Autodesk Inventor part; units mm, degrees
(part 4 of 6)
sketch "スケッチ4" plane through (0, 0, 3) normal (0, 0, 1) x (1, 0, 0)
  circle A0 centre (148.5, 105) radius 2 projected
  arc A1 (148.9109, 125.0429) -> (148.7771, 124.6719) centre (154.869, 122.6849) ccw projected
  arc A2 (149.1052, 125.4911) -> (148.9109, 125.0429) centre (155.9658, 122.2508) ccw projected
  arc A3 (149.5044, 125.4754) -> (149.1052, 125.4911) centre (148.5, 105) ccw projected
  arc A4 (149.6629, 125.0133) -> (149.5044, 125.4754) centre (142.4106, 122.7834) ccw projected
  arc A5 (149.7671, 124.633) -> (149.6629, 125.0133) centre (143.5382, 123.1301) ccw projected
  arc A6 (149.831, 124.3292) -> (149.7671, 124.633) centre (144.6423, 123.3965) ccw projected
  arc A7 (150.2091, 124.2995) -> (149.831, 124.3292) centre (148.5, 105) ccw projected
  arc A8 (150.3197, 124.5895) -> (150.2091, 124.2995) centre (155.1881, 122.5665) ccw projected
  arc A9 (150.4822, 124.9489) -> (150.3197, 124.5895) centre (156.2369, 122.1307) ccw projected
  arc A10 (150.7111, 125.3804) -> (150.4822, 124.9489) centre (157.2963, 121.6119) ccw projected
  arc A11 (151.1078, 125.3335) -> (150.7111, 125.3804) centre (148.5, 105) ccw projected
  arc A12 (151.2295, 124.8604) -> (151.1078, 125.3335) centre (143.8247, 123.2064) ccw projected
  arc A13 (151.3036, 124.473) -> (151.2295, 124.8604) centre (144.9759, 123.4635) ccw projected
  arc A14 (151.3435, 124.1652) -> (151.3036, 124.473) centre (146.0975, 123.6425) ccw projected
  arc A15 (151.7181, 124.1059) -> (151.3435, 124.1652) centre (148.5, 105) ccw projected
  arc A16 (151.8511, 124.3863) -> (151.7181, 124.1059) centre (156.5457, 121.9876) ccw projected
  arc A17 (152.0413, 124.7318) -> (151.8511, 124.3863) centre (157.5571, 121.4708) ccw projected
  arc A18 (152.3033, 125.1441) -> (152.0413, 124.7318) centre (158.5726, 120.8705) ccw projected
  arc A19 (152.6951, 125.0662) -> (152.3033, 125.1441) centre (148.5, 105) ccw projected
  arc A20 (152.7793, 124.585) -> (152.6951, 125.0662) centre (145.2676, 123.517) ccw projected
  arc A21 (152.8228, 124.193) -> (152.7793, 124.585) centre (146.4354, 123.6831) ccw projected
  arc A22 (152.8384, 123.883) -> (152.8228, 124.193) centre (147.5676, 123.7735) ccw projected
  arc A23 (153.2072, 123.7945) -> (152.8384, 123.883) centre (148.5, 105) ccw projected
  arc A24 (153.3618, 124.0636) -> (153.2072, 123.7945) centre (157.8537, 121.304) ccw projected
  arc A25 (153.5785, 124.3932) -> (153.3618, 124.0636) centre (158.8215, 120.7095) ccw projected
  arc A26 (153.872, 124.7836) -> (153.5785, 124.3932) centre (159.7867, 120.0313) ccw projected
  arc A27 (154.2565, 124.6752) -> (153.872, 124.7836) centre (148.5, 105) ccw projected
  arc A28 (154.3028, 124.1889) -> (154.2565, 124.6752) centre (146.7304, 123.7136) ccw projected
  arc A29 (154.3154, 123.7947) -> (154.3028, 124.1889) centre (147.9076, 123.7875) ccw projected
  arc A30 (154.3066, 123.4844) -> (154.3154, 123.7947) centre (149.0434, 123.7888) ccw projected
  arc A31 (154.6673, 123.3672) -> (154.3066, 123.4844) centre (148.5, 105) ccw projected
  arc A32 (154.8425, 123.6234) -> (154.6673, 123.3672) centre (159.1041, 120.5199) ccw projected
  arc A33 (155.0844, 123.9349) -> (154.8425, 123.6234) centre (160.0222, 119.8512) ccw projected
  arc A34 (155.4077, 124.3011) -> (155.0844, 123.9349) centre (160.9312, 119.0994) ccw projected
  arc A35 (155.7825, 124.1629) -> (155.4077, 124.3011) centre (148.5, 105) ccw projected
  arc A36 (155.7904, 123.6745) -> (155.7825, 124.1629) centre (148.2041, 123.7947) ccw projected
  arc A37 (155.772, 123.2805) -> (155.7904, 123.6745) centre (149.3835, 123.776) ccw projected
  arc A38 (155.7389, 122.9719) -> (155.772, 123.2805) centre (150.5159, 123.6882) ccw projected
  arc A39 (156.0893, 122.8267) -> (155.7389, 122.9719) centre (148.5, 105) ccw projected
  arc A40 (156.2842, 123.0684) -> (156.0893, 122.8267) centre (160.2891, 119.64) ccw projected
  arc A41 (156.5497, 123.36) -> (156.2842, 123.0684) centre (161.1519, 118.9014) ccw projected
  arc A42 (156.9007, 123.6997) -> (156.5497, 123.36) centre (161.9991, 118.0806) ccw projected
  arc A43 (157.2635, 123.5324) -> (156.9007, 123.6997) centre (148.5, 105) ccw projected
  arc A44 (157.2331, 123.0449) -> (157.2635, 123.5324) centre (149.6796, 123.76) ccw projected
  arc A45 (157.1839, 122.6536) -> (157.2331, 123.0449) centre (150.8539, 123.6488) ccw projected
  arc A46 (157.1267, 122.3485) -> (157.1839, 122.6536) centre (151.976, 123.4724) ccw projected
  arc A47 (157.4646, 122.1763) -> (157.1267, 122.3485) centre (148.5, 105) ccw projected
  arc A48 (157.6778, 122.4019) -> (157.4646, 122.1763) centre (161.4014, 118.6699) ccw projected
  arc A49 (157.9654, 122.6718) -> (157.6778, 122.4019) centre (162.2036, 117.8659) ccw projected
  arc A50 (158.342, 122.9829) -> (157.9654, 122.6718) centre (162.9838, 116.9812) ccw projected
  arc A51 (158.6905, 122.7877) -> (158.342, 122.9829) centre (148.5, 105) ccw projected
  arc A52 (158.622, 122.3041) -> (158.6905, 122.7877) centre (151.1478, 123.6096) ccw projected
  arc A53 (158.5422, 121.9178) -> (158.622, 122.3041) centre (152.3099, 123.4067) ccw projected
  arc A54 (158.4612, 121.6182) -> (158.5422, 121.9178) centre (153.4146, 123.1428) ccw projected
  arc A55 (158.7846, 121.42) -> (158.4612, 121.6182) centre (148.5, 105) ccw projected
  arc A56 (159.0148, 121.6282) -> (158.7846, 121.42) centre (162.4341, 117.6156) ccw projected
  arc A57 (159.3227, 121.8747) -> (159.0148, 121.6282) centre (163.1708, 116.7511) ccw projected
  arc A58 (159.7226, 122.1553) -> (159.3227, 121.8747) centre (163.8792, 115.8078) ccw projected
  arc A59 (160.0547, 121.9334) -> (159.7226, 122.1553) centre (148.5, 105) ccw projected
  arc A60 (159.9485, 121.4566) -> (160.0547, 121.9334) centre (152.5998, 123.3445) ccw projected
  arc A61 (159.8386, 121.0778) -> (159.9485, 121.4566) centre (153.7423, 123.051) ccw projected
  arc A62 (159.7344, 120.7854) -> (159.8386, 121.0778) centre (154.8229, 122.7012) ccw projected
  arc A63 (160.0412, 120.5625) -> (159.7344, 120.7854) centre (148.5, 105) ccw projected
  arc A64 (160.2871, 120.752) -> (160.0412, 120.5625) centre (163.381, 116.4834) ccw projected
  arc A65 (160.6134, 120.9735) -> (160.2871, 120.752) centre (164.0476, 115.5638) ccw projected
  arc A66 (161.034, 121.2219) -> (160.6134, 120.9735) centre (164.6798, 114.5679) ccw projected
  arc A67 (161.3477, 120.9746) -> (161.034, 121.2219) centre (148.5, 105) ccw projected
  arc A68 (161.2043, 120.5076) -> (161.3477, 120.9746) centre (154.0264, 122.9663) ccw projected
  arc A69 (161.0651, 120.1386) -> (161.2043, 120.5076) centre (155.1424, 122.5841) ccw projected
  arc A70 (160.9383, 119.8553) -> (161.0651, 120.1386) centre (156.1922, 122.1506) ccw projected
  arc A71 (161.2266, 119.609) -> (160.9383, 119.8553) centre (148.5, 105) ccw projected
  arc A72 (161.4866, 119.7786) -> (161.2266, 119.609) centre (164.2361, 115.2805) ccw projected
  arc A73 (161.8293, 119.9739) -> (161.4866, 119.7786) centre (164.8285, 114.3114) ccw projected
  arc A74 (162.2681, 120.1885) -> (161.8293, 119.9739) centre (165.3806, 113.2689) ccw projected
  arc A75 (162.5614, 119.9173) -> (162.2681, 120.1885) centre (148.5, 105) ccw projected
  arc A76 (162.3819, 119.463) -> (162.5614, 119.9173) centre (155.419, 122.4773) ccw projected
  arc A77 (162.2141, 119.1061) -> (162.3819, 119.463) centre (156.5015, 122.0087) ccw projected
  arc A78 (162.0655, 118.8336) -> (162.2141, 119.1061) centre (157.5141, 121.4942) ccw projected
  arc A79 (162.3336, 118.5655) -> (162.0655, 118.8336) centre (148.5, 105) ccw projected
  arc A80 (162.6061, 118.7141) -> (162.3336, 118.5655) centre (164.9942, 114.0141) ccw projected
  arc A81 (162.963, 118.8819) -> (162.6061, 118.7141) centre (165.5087, 113.0015) ccw projected
  arc A82 (163.4173, 119.0614) -> (162.963, 118.8819) centre (165.9773, 111.919) ccw projected
  arc A83 (163.6885, 118.7681) -> (163.4173, 119.0614) centre (148.5, 105) ccw projected
  arc A84 (163.4738, 118.3293) -> (163.6885, 118.7681) centre (156.7689, 121.8806) ccw projected
  arc A85 (163.2786, 117.9866) -> (163.4738, 118.3293) centre (157.8114, 121.3285) ccw projected
  arc A86 (163.109, 117.7266) -> (163.2786, 117.9866) centre (158.7805, 120.7361) ccw projected
  arc A87 (163.3553, 117.4383) -> (163.109, 117.7266) centre (148.5, 105) ccw projected
  arc A88 (163.6386, 117.5651) -> (163.3553, 117.4383) centre (165.6506, 112.6922) ccw projected
  arc A89 (164.0076, 117.7043) -> (163.6386, 117.5651) centre (166.0841, 111.6424) ccw projected
  arc A90 (164.4746, 117.8477) -> (164.0076, 117.7043) centre (166.4663, 110.5264) ccw projected
  arc A91 (164.7219, 117.534) -> (164.4746, 117.8477) centre (148.5, 105) ccw projected
  arc A92 (164.4735, 117.1134) -> (164.7219, 117.534) centre (158.0679, 121.1798) ccw projected
  arc A93 (164.252, 116.7871) -> (164.4735, 117.1134) centre (159.0638, 120.5476) ccw projected
  arc A94 (164.0625, 116.5412) -> (164.252, 116.7871) centre (159.9834, 119.881) ccw projected
  arc A95 (164.2854, 116.2344) -> (164.0625, 116.5412) centre (148.5, 105) ccw projected
  arc A96 (164.5778, 116.3386) -> (164.2854, 116.2344) centre (166.2012, 111.3229) ccw projected
  arc A97 (164.9566, 116.4485) -> (164.5778, 116.3386) centre (166.551, 110.2423) ccw projected
  arc A98 (165.4334, 116.5547) -> (164.9566, 116.4485) centre (166.8445, 109.0998) ccw projected
  arc A99 (165.6553, 116.2226) -> (165.4334, 116.5547) centre (148.5, 105) ccw projected
  arc A100 (165.3747, 115.8227) -> (165.6553, 116.2226) centre (159.3078, 120.3792) ccw projected
  arc A101 (165.1282, 115.5148) -> (165.3747, 115.8227) centre (160.2511, 119.6708) ccw projected
  arc A102 (164.92, 115.2846) -> (165.1282, 115.5148) centre (161.1156, 118.9341) ccw projected
  arc A103 (165.1182, 114.9612) -> (164.92, 115.2846) centre (148.5, 105) ccw projected
  arc A104 (165.4178, 115.0422) -> (165.1182, 114.9612) centre (166.6428, 109.9146) ccw projected
  arc A105 (165.8041, 115.122) -> (165.4178, 115.0422) centre (166.9067, 108.8099) ccw projected
  arc A106 (166.2877, 115.1905) -> (165.8041, 115.122) centre (167.1096, 107.6478) ccw projected
  arc A107 (166.4829, 114.842) -> (166.2877, 115.1905) centre (148.5, 105) ccw projected
  arc A108 (166.1718, 114.4654) -> (166.4829, 114.842) centre (160.4812, 119.4838) ccw projected
  arc A109 (165.9019, 114.1778) -> (166.1718, 114.4654) centre (161.3659, 118.7036) ccw projected
  arc A110 (165.6763, 113.9646) -> (165.9019, 114.1778) centre (162.1699, 117.9014) ccw projected
  arc A111 (165.8485, 113.6267) -> (165.6763, 113.9646) centre (148.5, 105) ccw projected
  arc A112 (166.1536, 113.6839) -> (165.8485, 113.6267) centre (166.9724, 108.476) ccw projected
  arc A113 (166.5449, 113.7331) -> (166.1536, 113.6839) centre (167.1488, 107.3539) ccw projected
  arc A114 (167.0324, 113.7635) -> (166.5449, 113.7331) centre (167.26, 106.1796) ccw projected
  arc A115 (167.1997, 113.4007) -> (167.0324, 113.7635) centre (148.5, 105) ccw projected
  arc A116 (166.86, 113.0497) -> (167.1997, 113.4007) centre (161.5806, 118.4991) ccw projected
  arc A117 (166.5684, 112.7842) -> (166.86, 113.0497) centre (162.4014, 117.6519) ccw projected
  arc A118 (166.3267, 112.5893) -> (166.5684, 112.7842) centre (163.14, 116.7891) ccw projected
  arc A119 (166.4719, 112.2389) -> (166.3267, 112.5893) centre (148.5, 105) ccw projected
  arc A120 (166.7805, 112.272) -> (166.4719, 112.2389) centre (167.1882, 107.0159) ccw projected
  arc A121 (167.1745, 112.2904) -> (166.7805, 112.272) centre (167.276, 105.8835) ccw projected
  arc A122 (167.6629, 112.2825) -> (167.1745, 112.2904) centre (167.2947, 104.7041) ccw projected
  arc A123 (167.8011, 111.9077) -> (167.6629, 112.2825) centre (148.5, 105) ccw projected
  arc A124 (167.4349, 111.5844) -> (167.8011, 111.9077) centre (162.5994, 117.4312) ccw projected
  arc A125 (167.1234, 111.3425) -> (167.4349, 111.5844) centre (163.3512, 116.5222) ccw projected
  arc A126 (166.8672, 111.1673) -> (167.1234, 111.3425) centre (164.0199, 115.6041) ccw projected
  arc A127 (166.9844, 110.8066) -> (166.8672, 111.1673) centre (148.5, 105) ccw projected
  arc A128 (167.2947, 110.8154) -> (166.9844, 110.8066) centre (167.2888, 105.5434) ccw projected
  arc A129 (167.6889, 110.8028) -> (167.2947, 110.8154) centre (167.2875, 104.4076) ccw projected
  arc A130 (168.1752, 110.7565) -> (167.6889, 110.8028) centre (167.2136, 103.2304) ccw projected
  arc A131 (168.2836, 110.372) -> (168.1752, 110.7565) centre (148.5, 105) ccw projected
  arc A132 (167.8932, 110.0785) -> (168.2836, 110.372) centre (163.5313, 116.2867) ccw projected
  arc A133 (167.5636, 109.8618) -> (167.8932, 110.0785) centre (164.2095, 115.3215) ccw projected
  arc A134 (167.2945, 109.7072) -> (167.5636, 109.8618) centre (164.804, 114.3537) ccw projected
  arc A135 (167.383, 109.3384) -> (167.2945, 109.7072) centre (148.5, 105) ccw projected
  arc A136 (167.693, 109.3228) -> (167.383, 109.3384) centre (167.2735, 104.0676) ccw projected
  arc A137 (168.085, 109.2793) -> (167.693, 109.3228) centre (167.1831, 102.9354) ccw projected
  arc A138 (168.5662, 109.1951) -> (168.085, 109.2793) centre (167.017, 101.7676) ccw projected
  arc A139 (168.6441, 108.8033) -> (168.5662, 109.1951) centre (148.5, 105) ccw projected
  arc A140 (168.2318, 108.5413) -> (168.6441, 108.8033) centre (164.3705, 115.0726) ccw projected
  arc A141 (167.8863, 108.3511) -> (168.2318, 108.5413) centre (164.9708, 114.0571) ccw projected
  arc A142 (167.6059, 108.2181) -> (167.8863, 108.3511) centre (165.4876, 113.0457) ccw projected
  arc A143 (167.6652, 107.8435) -> (167.6059, 108.2181) centre (148.5, 105) ccw projected
  arc A144 (167.973, 107.8036) -> (167.6652, 107.8435) centre (167.1425, 102.5975) ccw projected
  arc A145 (168.3604, 107.7295) -> (167.973, 107.8036) centre (166.9635, 101.4759) ccw projected
  arc A146 (168.8335, 107.6078) -> (168.3604, 107.7295) centre (166.7064, 100.3247) ccw projected
  arc A147 (168.8804, 107.2111) -> (168.8335, 107.6078) centre (148.5, 105) ccw projected
  arc A148 (168.4489, 106.9822) -> (168.8804, 107.2111) centre (165.1119, 113.7963) ccw projected
  arc A149 (168.0895, 106.8197) -> (168.4489, 106.9822) centre (165.6307, 112.7369) ccw projected
  arc A150 (167.7995, 106.7091) -> (168.0895, 106.8197) centre (166.0665, 111.6881) ccw projected
  arc A151 (167.8292, 106.331) -> (167.7995, 106.7091) centre (148.5, 105) ccw projected
  arc A152 (168.133, 106.2671) -> (167.8292, 106.331) centre (166.8965, 101.1423) ccw projected
  arc A153 (168.5133, 106.1629) -> (168.133, 106.2671) centre (166.6301, 100.0382) ccw projected
  arc A154 (168.9754, 106.0044) -> (168.5133, 106.1629) centre (166.2834, 98.9106) ccw projected
  arc A155 (168.9911, 105.6052) -> (168.9754, 106.0044) centre (148.5, 105) ccw projected
  arc A156 (168.5429, 105.4109) -> (168.9911, 105.6052) centre (165.7508, 112.4658) ccw projected
  arc A157 (168.1719, 105.2771) -> (168.5429, 105.4109) centre (166.1849, 111.369) ccw projected
  arc A158 (167.8741, 105.1896) -> (168.1719, 105.2771) centre (166.5371, 110.2892) ccw projected
  arc A159 (167.8741, 104.8104) -> (167.8741, 105.1896) centre (148.5, 105) ccw projected
  arc A160 (168.1719, 104.7229) -> (167.8741, 104.8104) centre (166.5371, 99.7108) ccw projected
  arc A161 (168.5429, 104.5891) -> (168.1719, 104.7229) centre (166.1849, 98.631) ccw projected
  arc A162 (168.9911, 104.3948) -> (168.5429, 104.5891) centre (165.7508, 97.5342) ccw projected
  arc A163 (168.9754, 103.9956) -> (168.9911, 104.3948) centre (148.5, 105) ccw projected
  arc A164 (168.5133, 103.8371) -> (168.9754, 103.9956) centre (166.2834, 111.0894) ccw projected
  arc A165 (168.133, 103.7329) -> (168.5133, 103.8371) centre (166.6301, 109.9618) ccw projected
  arc A166 (167.8292, 103.669) -> (168.133, 103.7329) centre (166.8965, 108.8577) ccw projected
  arc A167 (167.7995, 103.2909) -> (167.8292, 103.669) centre (148.5, 105) ccw projected
  arc A168 (168.0895, 103.1803) -> (167.7995, 103.2909) centre (166.0665, 98.3119) ccw projected
  arc A169 (168.4489, 103.0178) -> (168.0895, 103.1803) centre (165.6307, 97.2631) ccw projected
  arc A170 (168.8804, 102.7889) -> (168.4489, 103.0178) centre (165.1119, 96.2037) ccw projected
  arc A171 (168.8335, 102.3922) -> (168.8804, 102.7889) centre (148.5, 105) ccw projected
  arc A172 (168.3604, 102.2705) -> (168.8335, 102.3922) centre (166.7064, 109.6753) ccw projected
  arc A173 (167.973, 102.1964) -> (168.3604, 102.2705) centre (166.9635, 108.5241) ccw projected
  arc A174 (167.6652, 102.1565) -> (167.973, 102.1964) centre (167.1425, 107.4025) ccw projected
  arc A175 (167.6059, 101.7819) -> (167.6652, 102.1565) centre (148.5, 105) ccw projected
  arc A176 (167.8863, 101.6489) -> (167.6059, 101.7819) centre (165.4876, 96.9543) ccw projected
  arc A177 (168.2318, 101.4587) -> (167.8863, 101.6489) centre (164.9708, 95.9429) ccw projected
  arc A178 (168.6441, 101.1967) -> (168.2318, 101.4587) centre (164.3705, 94.9274) ccw projected
  arc A179 (168.5662, 100.8049) -> (168.6441, 101.1967) centre (148.5, 105) ccw projected
  arc A180 (168.085, 100.7207) -> (168.5662, 100.8049) centre (167.017, 108.2324) ccw projected
  arc A181 (167.693, 100.6772) -> (168.085, 100.7207) centre (167.1831, 107.0646) ccw projected
  arc A182 (167.383, 100.6616) -> (167.693, 100.6772) centre (167.2735, 105.9324) ccw projected
  arc A183 (167.2945, 100.2928) -> (167.383, 100.6616) centre (148.5, 105) ccw projected
  arc A184 (167.5636, 100.1382) -> (167.2945, 100.2928) centre (164.804, 95.6463) ccw projected
  arc A185 (167.8932, 99.9215) -> (167.5636, 100.1382) centre (164.2095, 94.6785) ccw projected
  arc A186 (168.2836, 99.628) -> (167.8932, 99.9215) centre (163.5313, 93.7133) ccw projected
  arc A187 (168.1752, 99.2435) -> (168.2836, 99.628) centre (148.5, 105) ccw projected
  arc A188 (167.6889, 99.1972) -> (168.1752, 99.2435) centre (167.2136, 106.7696) ccw projected
  arc A189 (167.2947, 99.1846) -> (167.6889, 99.1972) centre (167.2875, 105.5924) ccw projected
  arc A190 (166.9844, 99.1934) -> (167.2947, 99.1846) centre (167.2888, 104.4566) ccw projected
  arc A191 (166.8672, 98.8327) -> (166.9844, 99.1934) centre (148.5, 105) ccw projected
  arc A192 (167.1234, 98.6575) -> (166.8672, 98.8327) centre (164.0199, 94.3959) ccw projected
  arc A193 (167.4349, 98.4156) -> (167.1234, 98.6575) centre (163.3512, 93.4778) ccw projected
  arc A194 (167.8011, 98.0923) -> (167.4349, 98.4156) centre (162.5994, 92.5688) ccw projected
  arc A195 (167.6629, 97.7175) -> (167.8011, 98.0923) centre (148.5, 105) ccw projected
  arc A196 (167.1745, 97.7096) -> (167.6629, 97.7175) centre (167.2947, 105.2959) ccw projected
  arc A197 (166.7805, 97.728) -> (167.1745, 97.7096) centre (167.276, 104.1165) ccw projected
  arc A198 (166.4719, 97.7611) -> (166.7805, 97.728) centre (167.1882, 102.9841) ccw projected
  arc A199 (166.3267, 97.4107) -> (166.4719, 97.7611) centre (148.5, 105) ccw projected
  arc A200 (166.5684, 97.2158) -> (166.3267, 97.4107) centre (163.14, 93.2109) ccw projected
  arc A201 (166.86, 96.9503) -> (166.5684, 97.2158) centre (162.4014, 92.3481) ccw projected
  arc A202 (167.1997, 96.5993) -> (166.86, 96.9503) centre (161.5806, 91.5009) ccw projected
  arc A203 (167.0324, 96.2365) -> (167.1997, 96.5993) centre (148.5, 105) ccw projected
  arc A204 (166.5449, 96.2669) -> (167.0324, 96.2365) centre (167.26, 103.8204) ccw projected
  arc A205 (166.1536, 96.3161) -> (166.5449, 96.2669) centre (167.1488, 102.6461) ccw projected
  arc A206 (165.8485, 96.3733) -> (166.1536, 96.3161) centre (166.9724, 101.524) ccw projected
  arc A207 (165.6763, 96.0354) -> (165.8485, 96.3733) centre (148.5, 105) ccw projected
  arc A208 (165.9019, 95.8222) -> (165.6763, 96.0354) centre (162.1699, 92.0986) ccw projected
  arc A209 (166.1718, 95.5346) -> (165.9019, 95.8222) centre (161.3659, 91.2964) ccw projected
  arc A210 (166.4829, 95.158) -> (166.1718, 95.5346) centre (160.4812, 90.5162) ccw projected
  arc A211 (166.2877, 94.8095) -> (166.4829, 95.158) centre (148.5, 105) ccw projected
  arc A212 (165.8041, 94.878) -> (166.2877, 94.8095) centre (167.1096, 102.3522) ccw projected
  arc A213 (165.4178, 94.9578) -> (165.8041, 94.878) centre (166.9067, 101.1901) ccw projected
  arc A214 (165.1182, 95.0388) -> (165.4178, 94.9578) centre (166.6428, 100.0854) ccw projected
  arc A215 (164.92, 94.7154) -> (165.1182, 95.0388) centre (148.5, 105) ccw projected
  arc A216 (165.1282, 94.4852) -> (164.92, 94.7154) centre (161.1156, 91.0659) ccw projected
  arc A217 (165.3747, 94.1773) -> (165.1282, 94.4852) centre (160.2511, 90.3292) ccw projected
  arc A218 (165.6553, 93.7774) -> (165.3747, 94.1773) centre (159.3078, 89.6208) ccw projected
  arc A219 (165.4334, 93.4453) -> (165.6553, 93.7774) centre (148.5, 105) ccw projected
  arc A220 (164.9566, 93.5515) -> (165.4334, 93.4453) centre (166.8445, 100.9002) ccw projected
  arc A221 (164.5778, 93.6614) -> (164.9566, 93.5515) centre (166.551, 99.7577) ccw projected
  arc A222 (164.2854, 93.7656) -> (164.5778, 93.6614) centre (166.2012, 98.6771) ccw projected
  arc A223 (164.0625, 93.4588) -> (164.2854, 93.7656) centre (148.5, 105) ccw projected
  arc A224 (164.252, 93.2129) -> (164.0625, 93.4588) centre (159.9834, 90.119) ccw projected
  arc A225 (164.4735, 92.8866) -> (164.252, 93.2129) centre (159.0638, 89.4524) ccw projected
  arc A226 (164.7219, 92.466) -> (164.4735, 92.8866) centre (158.0679, 88.8202) ccw projected
  arc A227 (164.4746, 92.1523) -> (164.7219, 92.466) centre (148.5, 105) ccw projected
  arc A228 (164.0076, 92.2957) -> (164.4746, 92.1523) centre (166.4663, 99.4736) ccw projected
  arc A229 (163.6386, 92.4349) -> (164.0076, 92.2957) centre (166.0841, 98.3576) ccw projected
  arc A230 (163.3553, 92.5617) -> (163.6386, 92.4349) centre (165.6506, 97.3078) ccw projected
  arc A231 (163.109, 92.2734) -> (163.3553, 92.5617) centre (148.5, 105) ccw projected
  arc A232 (163.2786, 92.0134) -> (163.109, 92.2734) centre (158.7805, 89.2639) ccw projected
  arc A233 (163.4738, 91.6707) -> (163.2786, 92.0134) centre (157.8114, 88.6715) ccw projected
  arc A234 (163.6885, 91.2319) -> (163.4738, 91.6707) centre (156.7689, 88.1194) ccw projected
  arc A235 (163.4173, 90.9386) -> (163.6885, 91.2319) centre (148.5, 105) ccw projected
  arc A236 (162.963, 91.1181) -> (163.4173, 90.9386) centre (165.9773, 98.081) ccw projected
  arc A237 (162.6061, 91.2859) -> (162.963, 91.1181) centre (165.5087, 96.9985) ccw projected
  arc A238 (162.3336, 91.4345) -> (162.6061, 91.2859) centre (164.9942, 95.9859) ccw projected
  arc A239 (162.0655, 91.1664) -> (162.3336, 91.4345) centre (148.5, 105) ccw projected
  arc A240 (162.2141, 90.8939) -> (162.0655, 91.1664) centre (157.5141, 88.5058) ccw projected
  arc A241 (162.3819, 90.537) -> (162.2141, 90.8939) centre (156.5015, 87.9913) ccw projected
  arc A242 (162.5614, 90.0827) -> (162.3819, 90.537) centre (155.419, 87.5227) ccw projected
  arc A243 (162.2681, 89.8115) -> (162.5614, 90.0827) centre (148.5, 105) ccw projected
  arc A244 (161.8293, 90.0261) -> (162.2681, 89.8115) centre (165.3806, 96.7311) ccw projected
  arc A245 (161.4866, 90.2214) -> (161.8293, 90.0261) centre (164.8285, 95.6886) ccw projected
  arc A246 (161.2266, 90.391) -> (161.4866, 90.2214) centre (164.2361, 94.7195) ccw projected
  arc A247 (160.9383, 90.1447) -> (161.2266, 90.391) centre (148.5, 105) ccw projected
  arc A248 (161.0651, 89.8614) -> (160.9383, 90.1447) centre (156.1922, 87.8494) ccw projected
  arc A249 (161.2043, 89.4924) -> (161.0651, 89.8614) centre (155.1424, 87.4159) ccw projected
  arc A250 (161.3477, 89.0254) -> (161.2043, 89.4924) centre (154.0264, 87.0337) ccw projected
  arc A251 (161.034, 88.7781) -> (161.3477, 89.0254) centre (148.5, 105) ccw projected
  arc A252 (160.6134, 89.0265) -> (161.034, 88.7781) centre (164.6798, 95.4321) ccw projected
  arc A253 (160.2871, 89.248) -> (160.6134, 89.0265) centre (164.0476, 94.4362) ccw projected
  arc A254 (160.0412, 89.4375) -> (160.2871, 89.248) centre (163.381, 93.5166) ccw projected
  arc A255 (159.7344, 89.2146) -> (160.0412, 89.4375) centre (148.5, 105) ccw projected
  arc A256 (159.8386, 88.9222) -> (159.7344, 89.2146) centre (154.8229, 87.2988) ccw projected
  arc A257 (159.9485, 88.5434) -> (159.8386, 88.9222) centre (153.7423, 86.949) ccw projected
  arc A258 (160.0547, 88.0666) -> (159.9485, 88.5434) centre (152.5998, 86.6555) ccw projected
  arc A259 (159.7226, 87.8447) -> (160.0547, 88.0666) centre (148.5, 105) ccw projected
  arc A260 (159.3227, 88.1253) -> (159.7226, 87.8447) centre (163.8792, 94.1922) ccw projected
  arc A261 (159.0148, 88.3718) -> (159.3227, 88.1253) centre (163.1708, 93.2489) ccw projected
  arc A262 (158.7846, 88.58) -> (159.0148, 88.3718) centre (162.4341, 92.3844) ccw projected
  arc A263 (158.4612, 88.3818) -> (158.7846, 88.58) centre (148.5, 105) ccw projected
  arc A264 (158.5422, 88.0822) -> (158.4612, 88.3818) centre (153.4146, 86.8572) ccw projected
  arc A265 (158.622, 87.6959) -> (158.5422, 88.0822) centre (152.3099, 86.5933) ccw projected
  arc A266 (158.6905, 87.2123) -> (158.622, 87.6959) centre (151.1478, 86.3904) ccw projected
  arc A267 (158.342, 87.0171) -> (158.6905, 87.2123) centre (148.5, 105) ccw projected
  arc A268 (157.9654, 87.3282) -> (158.342, 87.0171) centre (162.9838, 93.0188) ccw projected
  arc A269 (157.6778, 87.5981) -> (157.9654, 87.3282) centre (162.2036, 92.1341) ccw projected
  arc A270 (157.4646, 87.8237) -> (157.6778, 87.5981) centre (161.4014, 91.3301) ccw projected
  arc A271 (157.1267, 87.6515) -> (157.4646, 87.8237) centre (148.5, 105) ccw projected
  arc A272 (157.1839, 87.3464) -> (157.1267, 87.6515) centre (151.976, 86.5276) ccw projected
  arc A273 (157.2331, 86.9551) -> (157.1839, 87.3464) centre (150.8539, 86.3512) ccw projected
  arc A274 (157.2635, 86.4676) -> (157.2331, 86.9551) centre (149.6796, 86.24) ccw projected
  arc A275 (156.9007, 86.3003) -> (157.2635, 86.4676) centre (148.5, 105) ccw projected
  arc A276 (156.5497, 86.64) -> (156.9007, 86.3003) centre (161.9991, 91.9194) ccw projected
  arc A277 (156.2842, 86.9316) -> (156.5497, 86.64) centre (161.1519, 91.0986) ccw projected
  arc A278 (156.0893, 87.1733) -> (156.2842, 86.9316) centre (160.2891, 90.36) ccw projected
  arc A279 (155.7389, 87.0281) -> (156.0893, 87.1733) centre (148.5, 105) ccw projected
  arc A280 (155.772, 86.7195) -> (155.7389, 87.0281) centre (150.5159, 86.3118) ccw projected
  arc A281 (155.7904, 86.3255) -> (155.772, 86.7195) centre (149.3835, 86.224) ccw projected
  arc A282 (155.7825, 85.8371) -> (155.7904, 86.3255) centre (148.2041, 86.2053) ccw projected
  arc A283 (155.4077, 85.6989) -> (155.7825, 85.8371) centre (148.5, 105) ccw projected
  arc A284 (155.0844, 86.0651) -> (155.4077, 85.6989) centre (160.9312, 90.9006) ccw projected
  arc A285 (154.8425, 86.3766) -> (155.0844, 86.0651) centre (160.0222, 90.1488) ccw projected
  arc A286 (154.6673, 86.6328) -> (154.8425, 86.3766) centre (159.1041, 89.4801) ccw projected
  arc A287 (154.3066, 86.5156) -> (154.6673, 86.6328) centre (148.5, 105) ccw projected
  arc A288 (154.3154, 86.2053) -> (154.3066, 86.5156) centre (149.0434, 86.2112) ccw projected
  arc A289 (154.3028, 85.8111) -> (154.3154, 86.2053) centre (147.9076, 86.2125) ccw projected
  arc A290 (154.2565, 85.3248) -> (154.3028, 85.8111) centre (146.7304, 86.2864) ccw projected
  arc A291 (153.872, 85.2164) -> (154.2565, 85.3248) centre (148.5, 105) ccw projected
  arc A292 (153.5785, 85.6068) -> (153.872, 85.2164) centre (159.7867, 89.9687) ccw projected
  arc A293 (153.3618, 85.9364) -> (153.5785, 85.6068) centre (158.8215, 89.2905) ccw projected
  arc A294 (153.2072, 86.2055) -> (153.3618, 85.9364) centre (157.8537, 88.696) ccw projected
  arc A295 (152.8384, 86.117) -> (153.2072, 86.2055) centre (148.5, 105) ccw projected
  arc A296 (152.8228, 85.807) -> (152.8384, 86.117) centre (147.5676, 86.2265) ccw projected
  arc A297 (152.7793, 85.415) -> (152.8228, 85.807) centre (146.4354, 86.3169) ccw projected
  arc A298 (152.6951, 84.9338) -> (152.7793, 85.415) centre (145.2676, 86.483) ccw projected
  arc A299 (152.3033, 84.8559) -> (152.6951, 84.9338) centre (148.5, 105) ccw projected
  arc A300 (152.0413, 85.2682) -> (152.3033, 84.8559) centre (158.5726, 89.1295) ccw projected
  arc A301 (151.8511, 85.6137) -> (152.0413, 85.2682) centre (157.5571, 88.5292) ccw projected
  arc A302 (151.7181, 85.8941) -> (151.8511, 85.6137) centre (156.5457, 88.0124) ccw projected
  arc A303 (151.3435, 85.8348) -> (151.7181, 85.8941) centre (148.5, 105) ccw projected
  arc A304 (151.3036, 85.527) -> (151.3435, 85.8348) centre (146.0975, 86.3575) ccw projected
  arc A305 (151.2295, 85.1396) -> (151.3036, 85.527) centre (144.9759, 86.5365) ccw projected
  arc A306 (151.1078, 84.6665) -> (151.2295, 85.1396) centre (143.8247, 86.7936) ccw projected
  arc A307 (150.7111, 84.6196) -> (151.1078, 84.6665) centre (148.5, 105) ccw projected
  arc A308 (150.4822, 85.0511) -> (150.7111, 84.6196) centre (157.2963, 88.3881) ccw projected
  arc A309 (150.3197, 85.4105) -> (150.4822, 85.0511) centre (156.2369, 87.8693) ccw projected
  arc A310 (150.2091, 85.7005) -> (150.3197, 85.4105) centre (155.1881, 87.4335) ccw projected
  arc A311 (149.831, 85.6708) -> (150.2091, 85.7005) centre (148.5, 105) ccw projected
  arc A312 (149.7671, 85.367) -> (149.831, 85.6708) centre (144.6423, 86.6035) ccw projected
  arc A313 (149.6629, 84.9867) -> (149.7671, 85.367) centre (143.5382, 86.8699) ccw projected
  arc A314 (149.5044, 84.5246) -> (149.6629, 84.9867) centre (142.4106, 87.2166) ccw projected
  arc A315 (149.1052, 84.5089) -> (149.5044, 84.5246) centre (148.5, 105) ccw projected
  arc A316 (148.9109, 84.9571) -> (149.1052, 84.5089) centre (155.9658, 87.7492) ccw projected
  arc A317 (148.7771, 85.3281) -> (148.9109, 84.9571) centre (154.869, 87.3151) ccw projected
  arc A318 (148.6896, 85.6259) -> (148.7771, 85.3281) centre (153.7892, 86.9629) ccw projected
  arc A319 (148.3104, 85.6259) -> (148.6896, 85.6259) centre (148.5, 105) ccw projected
  arc A320 (148.2229, 85.3281) -> (148.3104, 85.6259) centre (143.2108, 86.9629) ccw projected
  arc A321 (148.0891, 84.9571) -> (148.2229, 85.3281) centre (142.131, 87.3151) ccw projected
  arc A322 (147.8948, 84.5089) -> (148.0891, 84.9571) centre (141.0342, 87.7492) ccw projected
  arc A323 (147.4956, 84.5246) -> (147.8948, 84.5089) centre (148.5, 105) ccw projected
  arc A324 (147.3371, 84.9867) -> (147.4956, 84.5246) centre (154.5894, 87.2166) ccw projected
  arc A325 (147.2329, 85.367) -> (147.3371, 84.9867) centre (153.4618, 86.8699) ccw projected
  arc A326 (147.169, 85.6708) -> (147.2329, 85.367) centre (152.3577, 86.6035) ccw projected
  arc A327 (146.7909, 85.7005) -> (147.169, 85.6708) centre (148.5, 105) ccw projected
  arc A328 (146.6803, 85.4105) -> (146.7909, 85.7005) centre (141.8119, 87.4335) ccw projected
  arc A329 (146.5178, 85.0511) -> (146.6803, 85.4105) centre (140.7631, 87.8693) ccw projected
  arc A330 (146.2889, 84.6196) -> (146.5178, 85.0511) centre (139.7037, 88.3881) ccw projected
  arc A331 (145.8922, 84.6665) -> (146.2889, 84.6196) centre (148.5, 105) ccw projected
  arc A332 (145.7705, 85.1396) -> (145.8922, 84.6665) centre (153.1753, 86.7936) ccw projected
  arc A333 (145.6964, 85.527) -> (145.7705, 85.1396) centre (152.0241, 86.5365) ccw projected
  arc A334 (145.6565, 85.8348) -> (145.6964, 85.527) centre (150.9025, 86.3575) ccw projected
  arc A335 (145.2819, 85.8941) -> (145.6565, 85.8348) centre (148.5, 105) ccw projected
  arc A336 (145.1489, 85.6137) -> (145.2819, 85.8941) centre (140.4543, 88.0124) ccw projected
  arc A337 (144.9587, 85.2682) -> (145.1489, 85.6137) centre (139.4429, 88.5292) ccw projected
  arc A338 (144.6967, 84.8559) -> (144.9587, 85.2682) centre (138.4274, 89.1295) ccw projected
  arc A339 (144.3049, 84.9338) -> (144.6967, 84.8559) centre (148.5, 105) ccw projected
  arc A340 (144.2207, 85.415) -> (144.3049, 84.9338) centre (151.7324, 86.483) ccw projected
  arc A341 (144.1772, 85.807) -> (144.2207, 85.415) centre (150.5646, 86.3169) ccw projected
  arc A342 (144.1616, 86.117) -> (144.1772, 85.807) centre (149.4324, 86.2265) ccw projected
  arc A343 (143.7928, 86.2055) -> (144.1616, 86.117) centre (148.5, 105) ccw projected
  arc A344 (143.6382, 85.9364) -> (143.7928, 86.2055) centre (139.1463, 88.696) ccw projected
  arc A345 (143.4215, 85.6068) -> (143.6382, 85.9364) centre (138.1785, 89.2905) ccw projected
  arc A346 (143.128, 85.2164) -> (143.4215, 85.6068) centre (137.2133, 89.9687) ccw projected
  arc A347 (142.7435, 85.3248) -> (143.128, 85.2164) centre (148.5, 105) ccw projected
  arc A348 (142.6972, 85.8111) -> (142.7435, 85.3248) centre (150.2696, 86.2864) ccw projected
  arc A349 (142.6846, 86.2053) -> (142.6972, 85.8111) centre (149.0924, 86.2125) ccw projected
  arc A350 (142.6934, 86.5156) -> (142.6846, 86.2053) centre (147.9566, 86.2112) ccw projected
  arc A351 (142.3327, 86.6328) -> (142.6934, 86.5156) centre (148.5, 105) ccw projected
  arc A352 (142.1575, 86.3766) -> (142.3327, 86.6328) centre (137.8959, 89.4801) ccw projected
  arc A353 (141.9156, 86.0651) -> (142.1575, 86.3766) centre (136.9778, 90.1488) ccw projected
  arc A354 (141.5923, 85.6989) -> (141.9156, 86.0651) centre (136.0688, 90.9006) ccw projected
  arc A355 (141.2175, 85.8371) -> (141.5923, 85.6989) centre (148.5, 105) ccw projected
  arc A356 (141.2096, 86.3255) -> (141.2175, 85.8371) centre (148.7959, 86.2053) ccw projected
  arc A357 (141.228, 86.7195) -> (141.2096, 86.3255) centre (147.6165, 86.224) ccw projected
  arc A358 (141.2611, 87.0281) -> (141.228, 86.7195) centre (146.4841, 86.3118) ccw projected
  arc A359 (140.9107, 87.1733) -> (141.2611, 87.0281) centre (148.5, 105) ccw projected
  arc A360 (140.7158, 86.9316) -> (140.9107, 87.1733) centre (136.7109, 90.36) ccw projected
  arc A361 (140.4503, 86.64) -> (140.7158, 86.9316) centre (135.8481, 91.0986) ccw projected
  arc A362 (140.0993, 86.3003) -> (140.4503, 86.64) centre (135.0009, 91.9194) ccw projected
  arc A363 (139.7365, 86.4676) -> (140.0993, 86.3003) centre (148.5, 105) ccw projected
  arc A364 (139.7669, 86.9551) -> (139.7365, 86.4676) centre (147.3204, 86.24) ccw projected
  arc A365 (139.8161, 87.3464) -> (139.7669, 86.9551) centre (146.1461, 86.3512) ccw projected
  arc A366 (139.8733, 87.6515) -> (139.8161, 87.3464) centre (145.024, 86.5276) ccw projected
  arc A367 (139.5354, 87.8237) -> (139.8733, 87.6515) centre (148.5, 105) ccw projected
  arc A368 (139.3222, 87.5981) -> (139.5354, 87.8237) centre (135.5986, 91.3301) ccw projected
  arc A369 (139.0346, 87.3282) -> (139.3222, 87.5981) centre (134.7964, 92.1341) ccw projected
  arc A370 (138.658, 87.0171) -> (139.0346, 87.3282) centre (134.0162, 93.0188) ccw projected
  arc A371 (138.3095, 87.2123) -> (138.658, 87.0171) centre (148.5, 105) ccw projected
  arc A372 (138.378, 87.6959) -> (138.3095, 87.2123) centre (145.8522, 86.3904) ccw projected
  arc A373 (138.4578, 88.0822) -> (138.378, 87.6959) centre (144.6901, 86.5933) ccw projected
  arc A374 (138.5388, 88.3818) -> (138.4578, 88.0822) centre (143.5854, 86.8572) ccw projected
  arc A375 (138.2154, 88.58) -> (138.5388, 88.3818) centre (148.5, 105) ccw projected
  arc A376 (137.9852, 88.3718) -> (138.2154, 88.58) centre (134.5659, 92.3844) ccw projected
  arc A377 (137.6773, 88.1253) -> (137.9852, 88.3718) centre (133.8292, 93.2489) ccw projected
  arc A378 (137.2774, 87.8447) -> (137.6773, 88.1253) centre (133.1208, 94.1922) ccw projected
  arc A379 (136.9453, 88.0666) -> (137.2774, 87.8447) centre (148.5, 105) ccw projected
  arc A380 (137.0515, 88.5434) -> (136.9453, 88.0666) centre (144.4002, 86.6555) ccw projected
  arc A381 (137.1614, 88.9222) -> (137.0515, 88.5434) centre (143.2577, 86.949) ccw projected
  arc A382 (137.2656, 89.2146) -> (137.1614, 88.9222) centre (142.1771, 87.2988) ccw projected
  arc A383 (136.9588, 89.4375) -> (137.2656, 89.2146) centre (148.5, 105) ccw projected
  arc A384 (136.7129, 89.248) -> (136.9588, 89.4375) centre (133.619, 93.5166) ccw projected
  arc A385 (136.3866, 89.0265) -> (136.7129, 89.248) centre (132.9524, 94.4362) ccw projected
  arc A386 (135.966, 88.7781) -> (136.3866, 89.0265) centre (132.3202, 95.4321) ccw projected
  arc A387 (135.6523, 89.0254) -> (135.966, 88.7781) centre (148.5, 105) ccw projected
  arc A388 (135.7957, 89.4924) -> (135.6523, 89.0254) centre (142.9736, 87.0337) ccw projected
  arc A389 (135.9349, 89.8614) -> (135.7957, 89.4924) centre (141.8576, 87.4159) ccw projected
  arc A390 (136.0617, 90.1447) -> (135.9349, 89.8614) centre (140.8078, 87.8494) ccw projected
  arc A391 (135.7734, 90.391) -> (136.0617, 90.1447) centre (148.5, 105) ccw projected
  arc A392 (135.5134, 90.2214) -> (135.7734, 90.391) centre (132.7639, 94.7195) ccw projected
  arc A393 (135.1707, 90.0261) -> (135.5134, 90.2214) centre (132.1715, 95.6886) ccw projected
  arc A394 (134.7319, 89.8115) -> (135.1707, 90.0261) centre (131.6194, 96.7311) ccw projected
  arc A395 (134.4386, 90.0827) -> (134.7319, 89.8115) centre (148.5, 105) ccw projected
  arc A396 (134.6181, 90.537) -> (134.4386, 90.0827) centre (141.581, 87.5227) ccw projected
  arc A397 (134.7859, 90.8939) -> (134.6181, 90.537) centre (140.4985, 87.9913) ccw projected
  arc A398 (134.9345, 91.1664) -> (134.7859, 90.8939) centre (139.4859, 88.5058) ccw projected
  arc A399 (134.6664, 91.4345) -> (134.9345, 91.1664) centre (148.5, 105) ccw projected
  arc A400 (134.3939, 91.2859) -> (134.6664, 91.4345) centre (132.0058, 95.9859) ccw projected
  arc A401 (134.037, 91.1181) -> (134.3939, 91.2859) centre (131.4913, 96.9985) ccw projected
  arc A402 (133.5827, 90.9386) -> (134.037, 91.1181) centre (131.0227, 98.081) ccw projected
  arc A403 (133.3115, 91.2319) -> (133.5827, 90.9386) centre (148.5, 105) ccw projected
  arc A404 (133.5261, 91.6707) -> (133.3115, 91.2319) centre (140.2311, 88.1194) ccw projected
  arc A405 (133.7214, 92.0134) -> (133.5261, 91.6707) centre (139.1886, 88.6715) ccw projected
  arc A406 (133.891, 92.2734) -> (133.7214, 92.0134) centre (138.2195, 89.2639) ccw projected
  arc A407 (133.6447, 92.5617) -> (133.891, 92.2734) centre (148.5, 105) ccw projected
  arc A408 (133.3614, 92.4349) -> (133.6447, 92.5617) centre (131.3494, 97.3078) ccw projected
  arc A409 (132.9924, 92.2957) -> (133.3614, 92.4349) centre (130.9159, 98.3576) ccw projected
  arc A410 (132.5254, 92.1523) -> (132.9924, 92.2957) centre (130.5337, 99.4736) ccw projected
  arc A411 (132.2781, 92.466) -> (132.5254, 92.1523) centre (148.5, 105) ccw projected
  arc A412 (132.5265, 92.8866) -> (132.2781, 92.466) centre (138.9321, 88.8202) ccw projected
  arc A413 (132.748, 93.2129) -> (132.5265, 92.8866) centre (137.9362, 89.4524) ccw projected
  arc A414 (132.9375, 93.4588) -> (132.748, 93.2129) centre (137.0166, 90.119) ccw projected
  arc A415 (132.7146, 93.7656) -> (132.9375, 93.4588) centre (148.5, 105) ccw projected
  arc A416 (132.4222, 93.6614) -> (132.7146, 93.7656) centre (130.7988, 98.6771) ccw projected
  arc A417 (132.0434, 93.5515) -> (132.4222, 93.6614) centre (130.449, 99.7577) ccw projected
  arc A418 (131.5666, 93.4453) -> (132.0434, 93.5515) centre (130.1555, 100.9002) ccw projected
  arc A419 (131.3447, 93.7774) -> (131.5666, 93.4453) centre (148.5, 105) ccw projected
  arc A420 (131.6253, 94.1773) -> (131.3447, 93.7774) centre (137.6922, 89.6208) ccw projected
  arc A421 (131.8718, 94.4852) -> (131.6253, 94.1773) centre (136.7489, 90.3292) ccw projected
  arc A422 (132.08, 94.7154) -> (131.8718, 94.4852) centre (135.8844, 91.0659) ccw projected
  arc A423 (131.8818, 95.0388) -> (132.08, 94.7154) centre (148.5, 105) ccw projected
  arc A424 (131.5822, 94.9578) -> (131.8818, 95.0388) centre (130.3572, 100.0854) ccw projected
  arc A425 (131.1959, 94.878) -> (131.5822, 94.9578) centre (130.0933, 101.1901) ccw projected
  arc A426 (130.7123, 94.8095) -> (131.1959, 94.878) centre (129.8904, 102.3522) ccw projected
  arc A427 (130.5171, 95.158) -> (130.7123, 94.8095) centre (148.5, 105) ccw projected
  arc A428 (130.8282, 95.5346) -> (130.5171, 95.158) centre (136.5188, 90.5162) ccw projected
  arc A429 (131.0981, 95.8222) -> (130.8282, 95.5346) centre (135.6341, 91.2964) ccw projected
  arc A430 (131.3237, 96.0354) -> (131.0981, 95.8222) centre (134.8301, 92.0986) ccw projected
  arc A431 (131.1515, 96.3733) -> (131.3237, 96.0354) centre (148.5, 105) ccw projected
  arc A432 (130.8464, 96.3161) -> (131.1515, 96.3733) centre (130.0276, 101.524) ccw projected
  arc A433 (130.4551, 96.2669) -> (130.8464, 96.3161) centre (129.8512, 102.6461) ccw projected
  arc A434 (129.9676, 96.2365) -> (130.4551, 96.2669) centre (129.74, 103.8204) ccw projected
  arc A435 (129.8003, 96.5993) -> (129.9676, 96.2365) centre (148.5, 105) ccw projected
  arc A436 (130.14, 96.9503) -> (129.8003, 96.5993) centre (135.4194, 91.5009) ccw projected
  arc A437 (130.4316, 97.2158) -> (130.14, 96.9503) centre (134.5986, 92.3481) ccw projected
  arc A438 (130.6733, 97.4107) -> (130.4316, 97.2158) centre (133.86, 93.2109) ccw projected
  arc A439 (130.5281, 97.7611) -> (130.6733, 97.4107) centre (148.5, 105) ccw projected
  arc A440 (130.2195, 97.728) -> (130.5281, 97.7611) centre (129.8118, 102.9841) ccw projected
  arc A441 (129.8255, 97.7096) -> (130.2195, 97.728) centre (129.724, 104.1165) ccw projected
  arc A442 (129.3371, 97.7175) -> (129.8255, 97.7096) centre (129.7053, 105.2959) ccw projected
  arc A443 (129.1989, 98.0923) -> (129.3371, 97.7175) centre (148.5, 105) ccw projected
  arc A444 (129.5651, 98.4156) -> (129.1989, 98.0923) centre (134.4006, 92.5688) ccw projected
  arc A445 (129.8766, 98.6575) -> (129.5651, 98.4156) centre (133.6488, 93.4778) ccw projected
  arc A446 (130.1328, 98.8327) -> (129.8766, 98.6575) centre (132.9801, 94.3959) ccw projected
  arc A447 (130.0156, 99.1934) -> (130.1328, 98.8327) centre (148.5, 105) ccw projected
  arc A448 (129.7053, 99.1846) -> (130.0156, 99.1934) centre (129.7112, 104.4566) ccw projected
  arc A449 (129.3111, 99.1972) -> (129.7053, 99.1846) centre (129.7125, 105.5924) ccw projected
  arc A450 (128.8248, 99.2435) -> (129.3111, 99.1972) centre (129.7864, 106.7696) ccw projected
  arc A451 (128.7164, 99.628) -> (128.8248, 99.2435) centre (148.5, 105) ccw projected
  arc A452 (129.1068, 99.9215) -> (128.7164, 99.628) centre (133.4687, 93.7133) ccw projected
  arc A453 (129.4364, 100.1382) -> (129.1068, 99.9215) centre (132.7905, 94.6785) ccw projected
  arc A454 (129.7055, 100.2928) -> (129.4364, 100.1382) centre (132.196, 95.6463) ccw projected
  arc A455 (129.617, 100.6616) -> (129.7055, 100.2928) centre (148.5, 105) ccw projected
  arc A456 (129.307, 100.6772) -> (129.617, 100.6616) centre (129.7265, 105.9324) ccw projected
  arc A457 (128.915, 100.7207) -> (129.307, 100.6772) centre (129.8169, 107.0646) ccw projected
  arc A458 (128.4338, 100.8049) -> (128.915, 100.7207) centre (129.983, 108.2324) ccw projected
  arc A459 (128.3559, 101.1967) -> (128.4338, 100.8049) centre (148.5, 105) ccw projected
  arc A460 (128.7682, 101.4587) -> (128.3559, 101.1967) centre (132.6295, 94.9274) ccw projected
  arc A461 (129.1137, 101.6489) -> (128.7682, 101.4587) centre (132.0292, 95.9429) ccw projected
  arc A462 (129.3941, 101.7819) -> (129.1137, 101.6489) centre (131.5124, 96.9543) ccw projected
  arc A463 (129.3348, 102.1565) -> (129.3941, 101.7819) centre (148.5, 105) ccw projected
  arc A464 (129.027, 102.1964) -> (129.3348, 102.1565) centre (129.8575, 107.4025) ccw projected
  arc A465 (128.6396, 102.2705) -> (129.027, 102.1964) centre (130.0365, 108.5241) ccw projected
  arc A466 (128.1665, 102.3922) -> (128.6396, 102.2705) centre (130.2936, 109.6753) ccw projected
  arc A467 (128.1196, 102.7889) -> (128.1665, 102.3922) centre (148.5, 105) ccw projected
  arc A468 (128.5511, 103.0178) -> (128.1196, 102.7889) centre (131.8881, 96.2037) ccw projected
  arc A469 (128.9105, 103.1803) -> (128.5511, 103.0178) centre (131.3693, 97.2631) ccw projected
  arc A470 (129.2005, 103.2909) -> (128.9105, 103.1803) centre (130.9335, 98.3119) ccw projected
  arc A471 (129.1708, 103.669) -> (129.2005, 103.2909) centre (148.5, 105) ccw projected
  arc A472 (128.867, 103.7329) -> (129.1708, 103.669) centre (130.1035, 108.8577) ccw projected
  arc A473 (128.4867, 103.8371) -> (128.867, 103.7329) centre (130.3699, 109.9618) ccw projected
  arc A474 (128.0246, 103.9956) -> (128.4867, 103.8371) centre (130.7166, 111.0894) ccw projected
  arc A475 (128.0089, 104.3948) -> (128.0246, 103.9956) centre (148.5, 105) ccw projected
  arc A476 (128.4571, 104.5891) -> (128.0089, 104.3948) centre (131.2492, 97.5342) ccw projected
  arc A477 (128.8281, 104.7229) -> (128.4571, 104.5891) centre (130.8151, 98.631) ccw projected
  arc A478 (129.1259, 104.8104) -> (128.8281, 104.7229) centre (130.4629, 99.7108) ccw projected
  arc A479 (129.1259, 105.1896) -> (129.1259, 104.8104) centre (148.5, 105) ccw projected
  arc A480 (128.8281, 105.2771) -> (129.1259, 105.1896) centre (130.4629, 110.2892) ccw projected
  arc A481 (128.4571, 105.4109) -> (128.8281, 105.2771) centre (130.8151, 111.369) ccw projected
  arc A482 (128.0089, 105.6052) -> (128.4571, 105.4109) centre (131.2492, 112.4658) ccw projected
  arc A483 (128.0246, 106.0044) -> (128.0089, 105.6052) centre (148.5, 105) ccw projected
  arc A484 (128.4867, 106.1629) -> (128.0246, 106.0044) centre (130.7166, 98.9106) ccw projected
  arc A485 (128.867, 106.2671) -> (128.4867, 106.1629) centre (130.3699, 100.0382) ccw projected
  arc A486 (129.1708, 106.331) -> (128.867, 106.2671) centre (130.1035, 101.1423) ccw projected
  arc A487 (129.2005, 106.7091) -> (129.1708, 106.331) centre (148.5, 105) ccw projected
  arc A488 (128.9105, 106.8197) -> (129.2005, 106.7091) centre (130.9335, 111.6881) ccw projected
  arc A489 (128.5511, 106.9822) -> (128.9105, 106.8197) centre (131.3693, 112.7369) ccw projected
  arc A490 (128.1196, 107.2111) -> (128.5511, 106.9822) centre (131.8881, 113.7963) ccw projected
  arc A491 (128.1665, 107.6078) -> (128.1196, 107.2111) centre (148.5, 105) ccw projected
  arc A492 (128.6396, 107.7295) -> (128.1665, 107.6078) centre (130.2936, 100.3247) ccw projected
  arc A493 (129.027, 107.8036) -> (128.6396, 107.7295) centre (130.0365, 101.4759) ccw projected
  arc A494 (129.3348, 107.8435) -> (129.027, 107.8036) centre (129.8575, 102.5975) ccw projected
  arc A495 (129.3941, 108.2181) -> (129.3348, 107.8435) centre (148.5, 105) ccw projected
  arc A496 (129.1137, 108.3511) -> (129.3941, 108.2181) centre (131.5124, 113.0457) ccw projected
  arc A497 (128.7682, 108.5413) -> (129.1137, 108.3511) centre (132.0292, 114.0571) ccw projected
  arc A498 (128.3559, 108.8033) -> (128.7682, 108.5413) centre (132.6295, 115.0726) ccw projected
  arc A499 (128.4338, 109.1951) -> (128.3559, 108.8033) centre (148.5, 105) ccw projected
  arc A500 (128.915, 109.2793) -> (128.4338, 109.1951) centre (129.983, 101.7676) ccw projected
  arc A501 (129.307, 109.3228) -> (128.915, 109.2793) centre (129.8169, 102.9354) ccw projected
  arc A502 (129.617, 109.3384) -> (129.307, 109.3228) centre (129.7265, 104.0676) ccw projected
  arc A503 (129.7055, 109.7072) -> (129.617, 109.3384) centre (148.5, 105) ccw projected
  arc A504 (129.4364, 109.8618) -> (129.7055, 109.7072) centre (132.196, 114.3537) ccw projected
  arc A505 (129.1068, 110.0785) -> (129.4364, 109.8618) centre (132.7905, 115.3215) ccw projected
  arc A506 (128.7164, 110.372) -> (129.1068, 110.0785) centre (133.4687, 116.2867) ccw projected
  arc A507 (128.8248, 110.7565) -> (128.7164, 110.372) centre (148.5, 105) ccw projected
  arc A508 (129.3111, 110.8028) -> (128.8248, 110.7565) centre (129.7864, 103.2304) ccw projected
  arc A509 (129.7053, 110.8154) -> (129.3111, 110.8028) centre (129.7125, 104.4076) ccw projected
  arc A510 (130.0156, 110.8066) -> (129.7053, 110.8154) centre (129.7112, 105.5434) ccw projected
  arc A511 (130.1328, 111.1673) -> (130.0156, 110.8066) centre (148.5, 105) ccw projected
  arc A512 (129.8766, 111.3425) -> (130.1328, 111.1673) centre (132.9801, 115.6041) ccw projected
  arc A513 (129.5651, 111.5844) -> (129.8766, 111.3425) centre (133.6488, 116.5222) ccw projected
  arc A514 (129.1989, 111.9077) -> (129.5651, 111.5844) centre (134.4006, 117.4312) ccw projected
  arc A515 (129.3371, 112.2825) -> (129.1989, 111.9077) centre (148.5, 105) ccw projected
  arc A516 (129.8255, 112.2904) -> (129.3371, 112.2825) centre (129.7053, 104.7041) ccw projected
  arc A517 (130.2195, 112.272) -> (129.8255, 112.2904) centre (129.724, 105.8835) ccw projected
  arc A518 (130.5281, 112.2389) -> (130.2195, 112.272) centre (129.8118, 107.0159) ccw projected
  arc A519 (130.6733, 112.5893) -> (130.5281, 112.2389) centre (148.5, 105) ccw projected
  arc A520 (130.4316, 112.7842) -> (130.6733, 112.5893) centre (133.86, 116.7891) ccw projected
  arc A521 (130.14, 113.0497) -> (130.4316, 112.7842) centre (134.5986, 117.6519) ccw projected
  arc A522 (129.8003, 113.4007) -> (130.14, 113.0497) centre (135.4194, 118.4991) ccw projected
  arc A523 (129.9676, 113.7635) -> (129.8003, 113.4007) centre (148.5, 105) ccw projected
  arc A524 (130.4551, 113.7331) -> (129.9676, 113.7635) centre (129.74, 106.1796) ccw projected
  arc A525 (130.8464, 113.6839) -> (130.4551, 113.7331) centre (129.8512, 107.3539) ccw projected
  arc A526 (131.1515, 113.6267) -> (130.8464, 113.6839) centre (130.0276, 108.476) ccw projected
  arc A527 (131.3237, 113.9646) -> (131.1515, 113.6267) centre (148.5, 105) ccw projected
  arc A528 (131.0981, 114.1778) -> (131.3237, 113.9646) centre (134.8301, 117.9014) ccw projected
  arc A529 (130.8282, 114.4654) -> (131.0981, 114.1778) centre (135.6341, 118.7036) ccw projected
  arc A530 (130.5171, 114.842) -> (130.8282, 114.4654) centre (136.5188, 119.4838) ccw projected
  arc A531 (130.7123, 115.1905) -> (130.5171, 114.842) centre (148.5, 105) ccw projected
  arc A532 (131.1959, 115.122) -> (130.7123, 115.1905) centre (129.8904, 107.6478) ccw projected
  arc A533 (131.5822, 115.0422) -> (131.1959, 115.122) centre (130.0933, 108.8099) ccw projected
  arc A534 (131.8818, 114.9612) -> (131.5822, 115.0422) centre (130.3572, 109.9146) ccw projected
  arc A535 (132.08, 115.2846) -> (131.8818, 114.9612) centre (148.5, 105) ccw projected
  arc A536 (131.8718, 115.5148) -> (132.08, 115.2846) centre (135.8844, 118.9341) ccw projected
  arc A537 (131.6253, 115.8227) -> (131.8718, 115.5148) centre (136.7489, 119.6708) ccw projected
  arc A538 (131.3447, 116.2226) -> (131.6253, 115.8227) centre (137.6922, 120.3792) ccw projected
  arc A539 (131.5666, 116.5547) -> (131.3447, 116.2226) centre (148.5, 105) ccw projected
  arc A540 (132.0434, 116.4485) -> (131.5666, 116.5547) centre (130.1555, 109.0998) ccw projected
  arc A541 (132.4222, 116.3386) -> (132.0434, 116.4485) centre (130.449, 110.2423) ccw projected
  arc A542 (132.7146, 116.2344) -> (132.4222, 116.3386) centre (130.7988, 111.3229) ccw projected
  arc A543 (132.9375, 116.5412) -> (132.7146, 116.2344) centre (148.5, 105) ccw projected
  arc A544 (132.748, 116.7871) -> (132.9375, 116.5412) centre (137.0166, 119.881) ccw projected
  arc A545 (132.5265, 117.1134) -> (132.748, 116.7871) centre (137.9362, 120.5476) ccw projected
  arc A546 (132.2781, 117.534) -> (132.5265, 117.1134) centre (138.9321, 121.1798) ccw projected
  arc A547 (132.5254, 117.8477) -> (132.2781, 117.534) centre (148.5, 105) ccw projected
  arc A548 (132.9924, 117.7043) -> (132.5254, 117.8477) centre (130.5337, 110.5264) ccw projected
  arc A549 (133.3614, 117.5651) -> (132.9924, 117.7043) centre (130.9159, 111.6424) ccw projected
  arc A550 (133.6447, 117.4383) -> (133.3614, 117.5651) centre (131.3494, 112.6922) ccw projected
  arc A551 (133.891, 117.7266) -> (133.6447, 117.4383) centre (148.5, 105) ccw projected
  arc A552 (133.7214, 117.9866) -> (133.891, 117.7266) centre (138.2195, 120.7361) ccw projected
  arc A553 (133.5261, 118.3293) -> (133.7214, 117.9866) centre (139.1886, 121.3285) ccw projected
  arc A554 (133.3115, 118.7681) -> (133.5261, 118.3293) centre (140.2311, 121.8806) ccw projected
  arc A555 (133.5827, 119.0614) -> (133.3115, 118.7681) centre (148.5, 105) ccw projected
  arc A556 (134.037, 118.8819) -> (133.5827, 119.0614) centre (131.0227, 111.919) ccw projected
  arc A557 (134.3939, 118.7141) -> (134.037, 118.8819) centre (131.4913, 113.0015) ccw projected
  arc A558 (134.6664, 118.5655) -> (134.3939, 118.7141) centre (132.0058, 114.0141) ccw projected
  arc A559 (134.9345, 118.8336) -> (134.6664, 118.5655) centre (148.5, 105) ccw projected
  arc A560 (134.7859, 119.1061) -> (134.9345, 118.8336) centre (139.4859, 121.4942) ccw projected
  arc A561 (134.6181, 119.463) -> (134.7859, 119.1061) centre (140.4985, 122.0087) ccw projected
  arc A562 (134.4386, 119.9173) -> (134.6181, 119.463) centre (141.581, 122.4773) ccw projected
  arc A563 (134.7319, 120.1885) -> (134.4386, 119.9173) centre (148.5, 105) ccw projected
  arc A564 (135.1707, 119.9739) -> (134.7319, 120.1885) centre (131.6194, 113.2689) ccw projected
  arc A565 (135.5134, 119.7786) -> (135.1707, 119.9739) centre (132.1715, 114.3114) ccw projected
  arc A566 (135.7734, 119.609) -> (135.5134, 119.7786) centre (132.7639, 115.2805) ccw projected
  arc A567 (136.0617, 119.8553) -> (135.7734, 119.609) centre (148.5, 105) ccw projected
  arc A568 (135.9349, 120.1386) -> (136.0617, 119.8553) centre (140.8078, 122.1506) ccw projected
  arc A569 (135.7957, 120.5076) -> (135.9349, 120.1386) centre (141.8576, 122.5841) ccw projected
  arc A570 (135.6523, 120.9746) -> (135.7957, 120.5076) centre (142.9736, 122.9663) ccw projected
  arc A571 (135.966, 121.2219) -> (135.6523, 120.9746) centre (148.5, 105) ccw projected
  arc A572 (136.3866, 120.9735) -> (135.966, 121.2219) centre (132.3202, 114.5679) ccw projected
  arc A573 (136.7129, 120.752) -> (136.3866, 120.9735) centre (132.9524, 115.5638) ccw projected
  arc A574 (136.9588, 120.5625) -> (136.7129, 120.752) centre (133.619, 116.4834) ccw projected
  arc A575 (137.2656, 120.7854) -> (136.9588, 120.5625) centre (148.5, 105) ccw projected
  arc A576 (137.1614, 121.0778) -> (137.2656, 120.7854) centre (142.1771, 122.7012) ccw projected
  arc A577 (137.0515, 121.4566) -> (137.1614, 121.0778) centre (143.2577, 123.051) ccw projected
  arc A578 (136.9453, 121.9334) -> (137.0515, 121.4566) centre (144.4002, 123.3445) ccw projected
  arc A579 (137.2774, 122.1553) -> (136.9453, 121.9334) centre (148.5, 105) ccw projected
  arc A580 (137.6773, 121.8747) -> (137.2774, 122.1553) centre (133.1208, 115.8078) ccw projected
  arc A581 (137.9852, 121.6282) -> (137.6773, 121.8747) centre (133.8292, 116.7511) ccw projected
  arc A582 (138.2154, 121.42) -> (137.9852, 121.6282) centre (134.5659, 117.6156) ccw projected
  arc A583 (138.5388, 121.6182) -> (138.2154, 121.42) centre (148.5, 105) ccw projected
  arc A584 (138.4578, 121.9178) -> (138.5388, 121.6182) centre (143.5854, 123.1428) ccw projected
  arc A585 (138.378, 122.3041) -> (138.4578, 121.9178) centre (144.6901, 123.4067) ccw projected
  arc A586 (138.3095, 122.7877) -> (138.378, 122.3041) centre (145.8522, 123.6096) ccw projected
  arc A587 (138.658, 122.9829) -> (138.3095, 122.7877) centre (148.5, 105) ccw projected
  arc A588 (139.0346, 122.6718) -> (138.658, 122.9829) centre (134.0162, 116.9812) ccw projected
  arc A589 (139.3222, 122.4019) -> (139.0346, 122.6718) centre (134.7964, 117.8659) ccw projected
  arc A590 (139.5354, 122.1763) -> (139.3222, 122.4019) centre (135.5986, 118.6699) ccw projected
  arc A591 (139.8733, 122.3485) -> (139.5354, 122.1763) centre (148.5, 105) ccw projected
  arc A592 (139.8161, 122.6536) -> (139.8733, 122.3485) centre (145.024, 123.4724) ccw projected
  arc A593 (139.7669, 123.0449) -> (139.8161, 122.6536) centre (146.1461, 123.6488) ccw projected